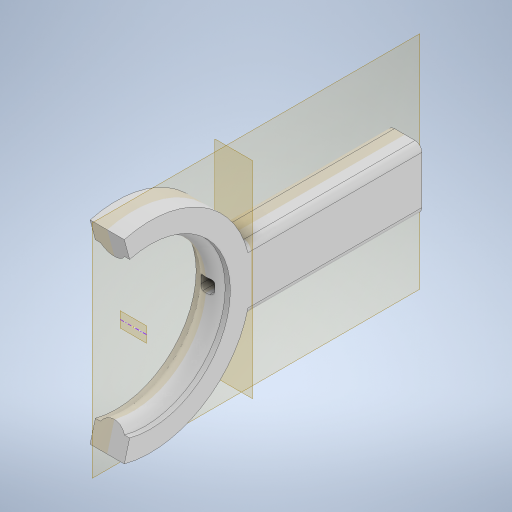
# Autodesk Inventor part: 막대대가리
Saved by Autodesk Inventor 2023 (Build 270158000, 158)
## iProperties
Created: 2023-04-26
Part Number: 막대대가리
Material: 일반
Document SubType Name: Modeling
Designer: rlatk
Density: 1 g/cm^3
Appearance: 기본값
Author: rlatk
Autodesk Inventor part; units mm, degrees
ref_plane "XZ Plane" through (0, 0, 0) normal (0, 1, 0) x (-1, 0, 0)
ref_plane "작업 평면1" through (0, 0, 11.4) normal (0, 0, 1) x (1, 0, 0)
sketch "스케치2" plane through (0, 0, 11.4) normal (0, 0, 1) x (1, 0, 0)
  line L0 (-3.8254, 0) -> (3.8254, 0)
  point P0 (0, 0)
  constraints: 2 end point, 1 horizontal
sketch "스케치1" plane through (0, 0, 0) normal (0, 1, 0) x (-1, 0, 0)
  line L0 (0, -12) -> (3.5, -12)
  line L1 (3.5, -12) -> (-3.5, -12)
  line L2 (0, -81.48) -> (0, 26.88) projected
  line L3 (0, -12) -> (0, -16)
  line L4 (0, -18) -> (5, -18)
  line L5 (5, -18) -> (5, -12)
  line L6 (5, -12) -> (3.5, -12)
  line L7 (0, -12) -> (-5, -12)
  line L8 (-5, -12) -> (-5, -18)
  arc A0 (3.5, -12) -> (-3.5, -12) centre (0, -13.9365) ccw
  line L9 (0, -18) -> (-5, -18)
  point P0 (0.0096, -9.9365)
  point P1 (0, -16)
  dimension "d0" = 3.5
  dimension "d1" = 3.5
  dimension "d60" = 4
  dimension "d61" = 5
  dimension "d62" = 6
  dimension "d63" = 5
  dimension "d64" = 6
  constraints: 18 end point, 3 point on circle, 1 centre point, 1 horizontal, 1 midpoint, 1 point on line, 1 other
  measures "d0" distance of L0.start L0.end
  measures "d1" distance of L0.start L1.end
  measures "d60" distance of L3.start L3.end
  measures "d61" distance of L4.start L4.end
  measures "d62" distance of L4.end L5.end
  measures "d63" distance of L3.start L7.end
  measures "d64" distance of L8.end L7.end
revolve "회전2" add sketch "스케치1" angle 105 about axis through (-3.8254, 0, 11.4) along (1, 0, 0) and the other way 105
ref_plane "작업 평면5" through (0, 0, -18) normal (0, 0, 1) x (1, 0, 0)
sketch "스케치20" plane through (0, 0, -18) normal (0, 0, 1) x (1, 0, 0)
  point P0 (0, 0)
sketch "스케치21" plane through (0, 0, -18) normal (0, 0, 1) x (1, 0, 0)
  point P0 (0, 0)
sketch "스케치22" plane through (0, 0, -18) normal (0, 0, 1) x (1, 0, 0)
  line L0 (-5, -29.4) -> (-5, 29.4) projected
  line L1 (-5, 9) -> (5, 9)
  line L2 (5, 9) -> (5, -9)
  line L3 (5, -9) -> (-5, -9)
  line L4 (-5, -9) -> (-5, 9)
  point P0 (0, 0)
  point P1 (-5, -28.3982)
  point P2 (-5, 28.3982)
  point P3 (-5, 0)
  dimension "d114" = 10
  dimension "d115" = 18
  constraints: 8 end point, 2 midpoint, 2 parallel, 1 horizontal, 1 perpendicular, 1 point on line
  measures "d114" distance of L2.end L3.end
  measures "d115" distance of L1.end L2.end
extrude "돌출20" add sketch "스케치22" against normal blind 50
sketch "스케치23" plane through (0, 0, 0) normal (1, 0, 0) x (0, 1, 0)
  line L0 (-9, -18) -> (0, -18) projected
  line L1 (-9, -18) -> (-9, -68) projected
  line L2 (9, -68) -> (-9, -68) projected
  line L3 (9, -18) -> (9, -68) projected
  line L4 (0, -18) -> (9, -18) projected
  line L5 (-22.6027, 17.4564) -> (-28.3982, 19.0093) projected
  arc A0 (-28.3982, 19.0093) -> (0, -18) centre (0, 11.4) ccw projected
  arc A1 (0, -18) -> (28.3982, 19.0093) centre (0, 11.4) ccw projected
  line L6 (22.6027, 17.4564) -> (28.3982, 19.0093) projected
  arc A2 (-22.6027, 17.4564) -> (22.6027, 17.4564) centre (0, 11.4) ccw projected
  line L7 (9, -18) -> (0, -18)
  arc A3 (-28.3982, 19.0093) -> (0, -18) centre (0, 11.4) ccw projected
  line L8 (0, -18) -> (-9, -18)
  line L9 (-9, -18) -> (-9, -16.5886)
  line L10 (9, -18) -> (9, -16.5886)
  arc A4 (0, -18) -> (9, -16.5886) centre (0, 11.4) ccw
  arc A5 (-9, -16.5886) -> (0, -18) centre (-0.3139, 9.3982) ccw
  point P0 (0, 0)
  point P1 (-9, -16.5886)
  point P2 (0, -18)
  point P3 (0, -18)
  point P4 (0, -18)
  point P5 (0, -18)
  constraints: 8 end point, 6 point on circle, 3 tangent, 2 centre point, 2 collinear, 1 concentric, 1 perpendicular, 1 vertical
extrude "돌출21" add sketch "스케치23" along normal blind 5 and the other way blind 5 contours A1 L10 L4 | L9 A5 L0
sketch "스케치24" plane through (0, 0, -68) normal (0, 0, -1) x (-1, 0, 0)
  line L0 (-2, -2) -> (2, -2)
  line L1 (2, -2) -> (2, 2)
  line L2 (2, 2) -> (-2, 2)
  line L3 (-2, 2) -> (-2, -2)
  line L4 (-5, 9) -> (-5, -9) projected
  line L5 (0, -41.16) -> (0, 41.16) projected
  point P0 (0, 0)
  point P1 (0, 2)
  dimension "d122" = 4
  dimension "d123" = 4
  constraints: 8 end point, 2 parallel, 1 horizontal, 1 midpoint, 1 perpendicular, 1 point on line
  measures "d122" distance of L2.end L1.end
  measures "d123" distance of L1.end L0.end
sketch "스케치25" plane through (0, 0, -68) normal (0, 0, -1) x (-1, 0, 0)
  point P0 (0, 0)
extrude "돌출22" cut sketch "스케치24" against normal blind 60
fillet "모깎기5" radius 2 4 edges at (5, -9, -42.2943) (-5, -9, -42.2943) (-5, 9, -42.2943) (5, 9, -42.2943)
fillet "모깎기6" radius 1 4 edges at (-2, -2, -39.1904) (2, -2, -39.1904) (-2, 2, -39.1904) (2, 2, -39.1904)
